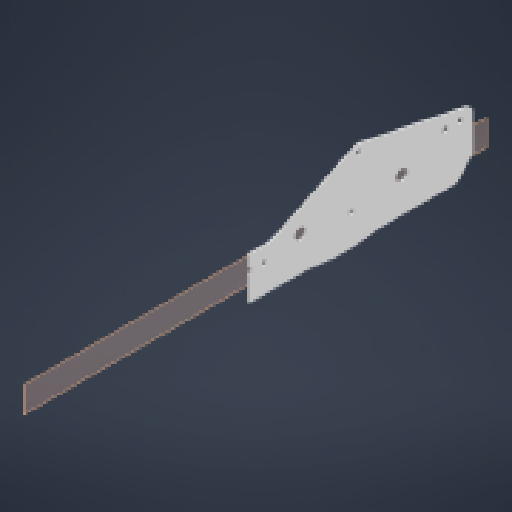
# Autodesk Inventor part: Part2
Saved by Autodesk Inventor 2026.1 (Build 301233000, 233)
## iProperties
Created: 2025-11-04
Part Number: Part2
Material: Generic
Document SubType Name: Modeling
Designer: jasper
Density: 1 g/cm^3
Appearance: Default
Author: jasper
Autodesk Inventor part; units mm, degrees
ref_plane "YZ Plane" through (0, 0, 0) normal (1, 0, 0) x (0, 1, 0)
ref_plane "XZ Plane" through (0, 0, 0) normal (0, 1, 0) x (-1, 0, 0)
ref_plane "XY Plane" through (0, 0, 0) normal (0, 0, 1) x (1, 0, 0)
ref_plane "Work Plane1" through (32.4184, 134.1094, 24.06) normal (1, 0, 0) x (0, 1, 0)
sketch "Sketch1" plane through (32.4184, 134.1094, 24.06) normal (1, 0, 0) x (0, 1, 0)
  line L0 (-24.13, 172.2574) -> (-24.13, 6.35) projected
  line L1 (-24.13, 6.35) -> (-2.1844, 6.35) projected
  line L2 (-10.3187, -184.15) -> (-2.3114, -184.15) projected
  circle A0 centre (6.35, -127) radius 2.1844 projected
  circle A1 centre (6.35, -38.1) radius 2.1844 projected
  circle A2 centre (0, -82.55) radius 2.1844 projected
  circle A3 centre (0, 6.35) radius 2.1844 projected
  circle A4 centre (0, -6.35) radius 2.1844 projected
  circle A5 centre (42.3182, -89.0797) radius 2.1844 projected
  line L3 (-24.13, 6.35) -> (-24.13, -172.0561)
  line L4 (-22.1107, -176.7002) -> (-10.5035, -187.5241)
  line L5 (-6.1728, -189.23) -> (22.9814, -189.23)
  line L6 (29.2006, -184.1621) -> (48.5374, -90.3617)
  line L7 (-24.13, 6.35) -> (12.7, 6.35)
  line L8 (12.7, -7.2898) -> (12.7, -68.7578) projected
  circle A6 centre (42.3182, -89.0797) radius 6.35
  line L9 (48.0429, -86.3318) -> (15.2013, -17.911)
  line L10 (12.7, -6.9198) -> (12.7, 6.35)
  circle A7 centre (21.8059, -177.8) radius 2.1844 projected
  circle A8 centre (21.8059, -165.1) radius 2.1844 projected
  arc A9 (12.7, -6.9198) -> (15.2013, -17.911) centre (38.1, -6.9198) ccw
  arc A10 (22.9814, -189.23) -> (29.2006, -184.1621) centre (22.9814, -182.88) ccw
  arc A11 (-10.5035, -187.5241) -> (-6.1728, -189.23) centre (-6.1728, -182.88) ccw
  arc A12 (-24.13, -172.0561) -> (-22.1107, -176.7002) centre (-17.78, -172.0561) ccw
  circle A13 centre (-6.35, -76.2) radius 2.1844 construction
  line L11 (-24.13, -40.64) -> (-24.13, -58.42) construction
  line L12 (-24.13, -58.42) -> (-32.512, -76.2) construction
  line L13 (-32.512, -76.2) -> (-24.13, -93.98) construction
  line L14 (-24.13, -93.98) -> (-24.13, -111.76) construction
  spline S0 degree 4 poles (-24.13, -40.64) (-24.13, -58.42) (-32.512, -76.2) (-24.13, -93.98) (-24.13, -111.76) knots 1 1 1 1 1 2 2 2 2 2
  circle A14 centre (6.35, -127) radius 4.953
  circle A15 centre (6.35, -38.1) radius 4.953
  circle A16 centre (0, -95.25) radius 2.1844
  point P0 (-134.1094, -24.06)
  point P1 (0, -82.55)
  point P2 (-8.6741, -189.23)
  point P3 (28.1559, -189.23)
  point P4 (12.7, -12.7)
  point P5 (-6.3151, -184.15)
  point P6 (2.1844, 6.35)
  point P7 (-24.13, -40.64)
  point P8 (-24.13, -111.76)
  dimension "d0" = 12.7
  dimension "d1" = 5.08
  dimension "d2" = 133
  dimension "d3" = 6.35
  dimension "d4" = 36.83
  dimension "d5" = 19.05
  dimension "d6" = 25.4
  dimension "d7" = 6.35
  dimension "d8" = 17.78
  dimension "d9" = 17.78
  dimension "d10" = 17.78
  dimension "d11" = 17.78
  dimension "d12" = 8.382
  dimension "d13" = 9.906
  dimension "d14" = 9.906
  dimension "d18" = 4.3688
  constraints: 14 end point, 10 point on circle, 10 tangent, 9 point on line, 8 centre point, 3 coincident, 3 vertical alignment, 2 equal radius, 1 collinear, 1 horizontal alignment, 1 midpoint, 1 perpendicular, 1 vertical, 5 other
  measures "d0" diameter of A6
  measures "d1" distance from line of point (-6.315, -184.15) L5
  measures "d2" angle of L3 L4
  measures "d3" horizontal distance of point (28.156, -189.23) A7.centre
  measures "d4" distance of point (-8.674, -189.23) point (28.156, -189.23)
  measures "d5" distance of point (12.7, -12.7) L7.end
  measures "d6" radius of A9
  measures "d7" radius of A10
  measures "d8" distance of L11.start L11.end
  measures "d9" distance of L13.end L14.end
  measures "d10" vertical distance of L12.end L13.end
  measures "d11" vertical distance of L11.end L12.end
  measures "d12" horizontal distance of L13.end L12.end
  measures "d13" diameter of A15
  measures "d14" diameter of A14
  measures "d18" diameter of A16
extrude "Extrusion1" add sketch "Sketch1" along normal blind 1.5875 contours L1 A3 L7 L10 A9 L9 A6 L6 A10 L5 A11 L4 A12 L3 | L3 S0 | A6 | A16
body "Solid1"
